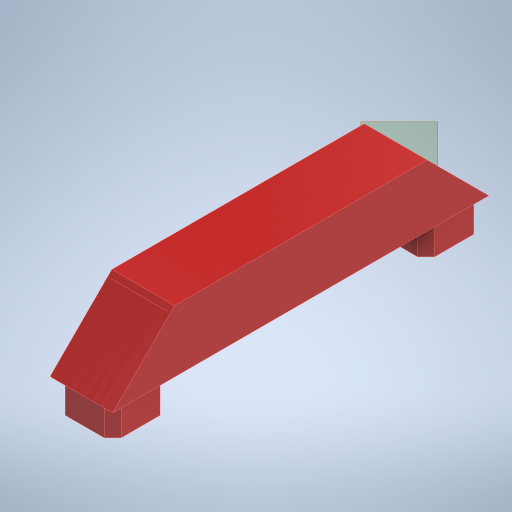
# Autodesk Inventor part: connector_part
Saved by Autodesk Inventor 2024 (Build 280153000, 153)
## iProperties
Created: 2024-04-21
Part Number: connector_part
Material: Rubber
Document SubType Name: Modeling
Designer: kamil
Density: 0.93 g/cm^3
Appearance: Red
Author: kamil
Autodesk Inventor part; units mm, degrees
ref_plane "YZ Plane" through (0, 0, 0) normal (1, 0, 0) x (0, 1, 0)
ref_plane "XZ Plane" through (0, 0, 0) normal (0, 1, 0) x (-1, 0, 0)
ref_plane "XY Plane" through (0, 0, 0) normal (0, 0, 1) x (1, 0, 0)
sketch "Sketch1" plane through (0, 0, 0) normal (0, 1, 0) x (-1, 0, 0)
  line L0 (75, 0) -> (0, 0)
  line L1 (0, 0) -> (0, -450)
  line L2 (0, -450) -> (75, -450)
  line L3 (75, -450) -> (75, 0)
  dimension "d0" = 450
  dimension "d1" = 75
  constraints: 8 end point, 2 parallel, 1 coincident, 1 horizontal, 1 perpendicular
  measures "d0" distance of L2.end L0.start
  measures "d1" distance of L1.end L2.end
extrude "Extrusion1" add sketch "Sketch1" along normal blind 4
sketch "Sketch2" plane through (0, 4, 0) normal (0, 1, 0) x (1, 0, 0)
  line L0 (-75, 450) -> (-75, 0) projected
  line L1 (0, 0) -> (-75, 0)
  line L2 (-75, 0) -> (-75, 450)
  line L3 (-75, 450) -> (0, 450)
  line L4 (0, 450) -> (0, 0)
  line L5 (-71, 446) -> (-71, 4)
  line L6 (-71, 4) -> (-4, 4)
  line L7 (-4, 4) -> (-4, 446)
  line L8 (-4, 446) -> (-71, 446)
  point P0 (-75, 0)
  dimension "d4" = 4
  constraints: 16 end point, 4 parallel, 2 perpendicular, 1 horizontal, 3 other
  measures "d4" distance between parallel lines of L2 L5
extrude "Extrusion2" add sketch "Sketch2" along normal blind 65
sketch "Sketch3" plane through (0, 69, 0) normal (0, 1, 0) x (1, 0, 0)
  line L0 (0, 0) -> (0, 450) projected
  line L1 (-75, 450) -> (-75, 0) projected
  line L2 (0, 0) -> (-75, 0)
  line L3 (-75, 0) -> (-75, 450)
  line L4 (-75, 450) -> (0, 450)
  line L5 (0, 450) -> (0, 0)
  point P0 (-75, 0)
  constraints: 8 end point, 2 parallel, 1 horizontal, 1 perpendicular
extrude "Extrusion3" add sketch "Sketch3" along normal blind 5
sketch "Sketch9" plane through (-75, 74, -450) normal (-1, 0, 0) x (0, 0, 1)
  line L0 (450, 0) -> (0, 0) projected
  line L1 (450, -74) -> (376, 0)
  line L2 (450, -74) -> (450, 0)
  line L3 (446, -70) -> (446, -5) projected
  line L4 (376, 0) -> (450, 0)
  line L5 (74.5, 0) -> (0, 0)
  line L6 (0, 0) -> (74.5, 0)
  line L7 (225, 0) -> (225, -74) construction
  line L8 (0, 0) -> (450, 0)
  line L9 (0, -74) -> (74, 0)
  line L10 (0, -74) -> (0, 0)
  point P0 (0, -149)
  dimension "d32" = 74
  constraints: 18 end point, 4 symmetric about line, 3 collinear, 3 point on line, 1 midpoint, 1 parallel, 1 vertical
  measures "d32" horizontal distance of L1.start L1.end
extrude "Extrusion8" cut sketch "Sketch9" against normal blind 75
sketch "Sketch10" plane through (0, 0, 0) normal (0, -1, 0) x (1, 0, 0)
  line L0 (-71, -4) -> (-4, -4) projected
  line L1 (-61, -4) -> (-14, -4)
  line L2 (-4, -14) -> (-4, -61)
  line L3 (-14, -71) -> (-61, -71)
  line L4 (-71, -61) -> (-71, -14)
  line L5 (-75, -450) -> (-75, 0) projected
  line L6 (-75, 0) -> (0, 0) projected
  line L7 (-75, -225) -> (0, -225) construction
  line L8 (0, -74) -> (0, -376) construction
  line L9 (-61, -446) -> (-14, -446)
  line L10 (-4, -436) -> (-4, -389)
  line L11 (-14, -379) -> (-61, -379)
  line L12 (-71, -389) -> (-71, -436)
  line L13 (-71, -61) -> (-61, -71)
  line L14 (-14, -71) -> (-4, -61)
  line L15 (-4, -14) -> (-14, -4)
  line L16 (-61, -4) -> (-71, -14)
  line L17 (-71, -436) -> (-61, -446)
  line L18 (-4, -436) -> (-14, -446)
  line L19 (-14, -379) -> (-4, -389)
  line L20 (-71, -389) -> (-61, -379)
  point P0 (-4, -71)
  point P1 (-4, -4)
  point P2 (-71, -71)
  point P3 (-71, -446)
  point P4 (-4, -446)
  point P5 (-4, -379)
  point P6 (-4, -446)
  point P7 (-71, -379)
  point P8 (-4, -446)
  point P9 (-4, -446)
  dimension "d37" = 67
  dimension "d38" = 67
  dimension "d39" = 4
  dimension "d40" = 4
  dimension "d43" = 10
  dimension "d44" = 10
  dimension "d45" = 10
  dimension "d46" = 10
  dimension "d47" = 10
  dimension "d48" = 10
  dimension "d49" = 10
  dimension "d50" = 10
  dimension "d51" = 10
  dimension "d52" = 10
  dimension "d53" = 10
  dimension "d54" = 10
  dimension "d55" = 10
  dimension "d56" = 10
  dimension "d57" = 10
  dimension "d58" = 10
  constraints: 34 end point, 18 point on line, 5 symmetric about line, 2 midpoint, 2 parallel, 1 horizontal, 1 perpendicular
  measures "d37" distance of point (-4, -71) point (-71, -71)
  measures "d38" distance of point (-4, -4) point (-4, -71)
  measures "d39" distance between parallel lines of L5 L4
  measures "d40" distance between parallel lines of L6 L0
  measures "d43" distance of L4.start point (-71, -71)
  measures "d44" distance of L3.end point (-71, -71)
  measures "d45" distance of L3.start point (-4, -71)
  measures "d46" distance of L2.end point (-4, -71)
  measures "d47" distance of L2.start point (-4, -4)
  measures "d48" distance of L1.end point (-4, -4)
  measures "d49" distance of L1.start L0.start
  measures "d50" distance of L4.end L0.start
  measures "d51" distance of L12.end point (-71, -446)
  measures "d52" distance of L9.start point (-71, -446)
  measures "d53" distance of L10.start point (-4, -446)
  measures "d54" distance of L9.end point (-4, -446)
  measures "d55" distance of L11.start point (-4, -379)
  measures "d56" distance of L10.end point (-4, -379)
  measures "d57" distance of L12.start point (-71, -379)
  measures "d58" distance of L11.end point (-71, -379)
extrude "Extrusion9" add sketch "Sketch10" along normal blind 35
sketch "Sketch11" plane through (-75, 0, 0) normal (0, 0.7071068, 0.7071068) x (1, 0, 0)
  line L0 (71, 97.5807) -> (4, 97.5807) projected
  line L1 (71, 5.6569) -> (71, 318.1981) projected
  line L2 (4, 97.5807) -> (71, 97.5807)
  line L3 (71, 97.5807) -> (71, 5.6569)
  line L4 (71, 5.6569) -> (4, 5.6569)
  line L5 (4, 5.6569) -> (4, 97.5807)
  point P0 (75, 0)
  constraints: 8 end point, 2 parallel, 1 horizontal, 1 perpendicular
extrude "Extrusion10" add sketch "Sketch11" against normal blind 4
sketch "Sketch12" plane through (0, 0, -450) normal (0, 0.7071068, -0.7071068) x (-1, 0, 0)
  line L0 (71, 97.5807) -> (4, 97.5807) projected
  line L1 (4, 5.6569) -> (71, 5.6569) projected
  line L2 (4, 97.5807) -> (71, 97.5807)
  line L3 (71, 97.5807) -> (71, 5.6569)
  line L4 (71, 5.6569) -> (4, 5.6569)
  line L5 (4, 5.6569) -> (4, 97.5807)
  point P0 (0, 318.1981)
  constraints: 8 end point, 2 parallel, 1 horizontal, 1 perpendicular
extrude "Extrusion11" add sketch "Sketch12" against normal blind 4
sketch "Sketch14" plane through (0, 0, 0) normal (0, -1, 0) x (1, 0, 0)
  line L0 (0, -450) -> (-75, -450) projected
  line L1 (-65.1005, -450) -> (-75, -440.1005)
  line L2 (-75, -376) -> (-75, -450) projected
  line L3 (-65.1005, -450) -> (-75, -450)
  line L4 (-75, -440.1005) -> (-75, -450)
  point P0 (0, 0)
  dimension "d64" = 45
  dimension "d65" = 14
  constraints: 6 end point, 2 point on line, 1 collinear, 1 perpendicular
  measures "d64" angle of L0 L1
  measures "d65" distance of L1.start L1.end
extrude "Extrusion12" cut sketch "Sketch14" against normal blind 10
sketch "Sketch19" plane through (-75, 74, -376) normal (-1, 0, 0) x (0, 0, 1)
  point P0 (376, -74)
ref_plane "Work Plane1" through (-65.1005, 0, -450) normal (-0.6029852, 0.5223196, -0.6029852) x (-0.7071068, 0, 0.7071068)
sketch "Sketch20" plane through (-65.1005, 0, -450) normal (-0.6029852, 0.5223196, -0.6029852) x (-0.7071068, 0, 0.7071068)
  line L0 (14, 0) -> (0, 0) projected
  line L1 (0, 0) -> (14, 0)
  line L2 (59.3259, 86.7781) -> (272.8721, 198.3175) projected
  line L3 (14, 0) -> (59.3259, 86.7781)
  line L4 (59.3259, 86.7781) -> (0, 0)
  point P0 (272.165, 190.245)
  constraints: 6 end point, 1 collinear
extrude "Extrusion13" cut sketch "Sketch20" along normal blind 10
equation "\"d44\" = d43"
equation "\"d45\" = d43"
equation "\"d46\" = d45"
equation "\"d47\" = d43"
equation "\"d48\" = d47"
equation "\"d49\" = d43"
equation "\"d50\" = d49"
equation "\"d51\" = d43"
equation "\"d52\" = d51"
equation "\"d53\" = d43"
equation "\"d54\" = d53"
equation "\"d55\" = d43"
equation "\"d56\" = d55"
equation "\"d57\" = d43"
equation "\"d58\" = d57"
body "Solid1"
